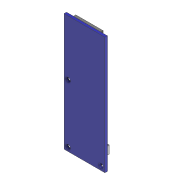
# Autodesk Inventor part: ESP32
Saved by Autodesk Inventor 2022.3 (Build 263350000, 350)
## iProperties
Created: 2023-07-18
Part Number: ESP32
Material: Genérico
Document SubType Name: Modeling
Designer: Usuario
Density: 1 g/cm^3
Appearance: Valor por defecto
Author: Usuario
Autodesk Inventor part; units mm, degrees
ref_plane "YZ Plane" through (0, 0, 0) normal (1, 0, 0) x (0, 1, 0)
ref_plane "XZ Plane" through (0, 0, 0) normal (0, 1, 0) x (-1, 0, 0)
ref_plane "XY Plane" through (0, 0, 0) normal (0, 0, 1) x (1, 0, 0)
sketch "Boceto1" plane through (0, 0, 0) normal (0, 0, 1) x (1, 0, 0)
  line L0 (-13.125, -37.65) -> (13.125, -37.65)
  line L1 (13.125, -37.65) -> (13.125, 37.65)
  line L2 (13.125, 37.65) -> (-13.125, 37.65)
  line L3 (-13.125, 37.65) -> (-13.125, -37.65)
  line L4 (-13.125, -37.65) -> (13.125, 37.65) construction
  line L5 (13.125, -37.65) -> (-13.125, 37.65) construction
  line L6 (0, -37.65) -> (0, -35.15)
  line L7 (0, -35.15) -> (10.5, -35.15)
  line L8 (10.5, -35.15) -> (-10.5, -35.15)
  circle A0 centre (10.5, -35.15) radius 1.5
  circle A1 centre (-10.5, -35.15) radius 1.5
  line L9 (-10.5, -35.15) -> (-10.5, 2.15)
  circle A2 centre (-10.5, 2.15) radius 1.5
  point P0 (0, 0)
  dimension "d0" = 26.25
  dimension "d1" = 75.3
  dimension "d2" = 2.5
  dimension "d3" = 10.5
  dimension "d4" = 21
  dimension "d5" = 3
  dimension "d6" = 3
  dimension "d7" = 37.3
  dimension "d8" = 3
  constraints: 20 end point, 3 centre point, 3 coincident, 3 midpoint, 3 perpendicular, 2 parallel, 1 horizontal, 1 point on line, 1 vertical
  measures "d0" distance of L2.end L1.end
  measures "d1" distance of L1.end L0.end
  measures "d2" distance of L6.start L6.end
  measures "d3" distance of L6.end L7.end
  measures "d4" distance of L7.end L8.end
  measures "d5" diameter of A0
  measures "d6" diameter of A1
  measures "d7" distance of L9.start L9.end
  measures "d8" diameter of A2
extrude "Extrusión1" add sketch "Boceto1" along normal blind 1.6
sketch "Boceto3" plane through (0, 0, 0) normal (0, 0, -1) x (-1, 0, 0)
  line L0 (-13.125, 37.65) -> (13.125, 37.65) projected
  line L1 (8.7698, 11.9975) -> (-8.7698, 11.9975)
  line L2 (-8.7698, 11.9975) -> (-8.7698, 37.65)
  line L3 (-8.7698, 37.65) -> (8.7698, 37.65)
  line L4 (8.7698, 37.65) -> (8.7698, 11.9975)
  line L5 (8.7698, 11.9975) -> (-8.7698, 37.65) construction
  line L6 (-8.7698, 11.9975) -> (8.7698, 37.65) construction
  line L7 (7.9072, -18.1146) -> (-7.9072, -18.1146)
  line L8 (-7.9072, -18.1146) -> (-7.9072, -2.2044)
  line L9 (-7.9072, -2.2044) -> (7.9072, -2.2044)
  line L10 (7.9072, -2.2044) -> (7.9072, -18.1146)
  line L11 (7.9072, -18.1146) -> (-7.9072, -2.2044) construction
  line L12 (-7.9072, -18.1146) -> (7.9072, -2.2044) construction
  point P0 (0, 0)
  point P1 (0, 24.8238)
  point P2 (0, -10.1595)
  constraints: 24 end point, 4 midpoint, 4 parallel, 2 horizontal, 2 perpendicular, 1 point on line
extrude "Extrusión2" add sketch "Boceto3" along normal blind 1.6
sketch "Boceto4" plane through (0, 0, -1.6) normal (0, 0, -1) x (-1, 0, 0)
  line L0 (8.003, 29.9035) -> (-8.003, 29.9035)
  line L1 (-8.003, 29.9035) -> (-8.003, 12.6515)
  line L2 (-8.003, 12.6515) -> (8.003, 12.6515)
  line L3 (8.003, 12.6515) -> (8.003, 29.9035)
  line L4 (8.003, 29.9035) -> (-8.003, 12.6515) construction
  line L5 (-8.003, 29.9035) -> (8.003, 12.6515) construction
  point P0 (0, 0)
  point P1 (0, 21.2775)
  constraints: 12 end point, 2 midpoint, 2 parallel, 1 horizontal, 1 perpendicular
extrude "Extrusión3" add sketch "Boceto4" along normal blind 2.5
sketch "Boceto5" plane through (-13.125, 37.65, 1.6) normal (0, 1, 0) x (1, 0, 0)
  line L0 (21.8948, 3.2) -> (4.3552, 3.2) projected
  line L1 (21.8948, 1.6) -> (21.8948, 3.2) projected
  line L2 (4.3552, 3.2) -> (21.8948, 3.2)
  line L3 (21.8948, 3.2) -> (21.8948, 1.6)
  line L4 (21.8948, 1.6) -> (4.3552, 1.6)
  line L5 (4.3552, 1.6) -> (4.3552, 3.2)
  point P0 (13.125, 1.6)
  constraints: 8 end point, 2 parallel, 1 horizontal, 1 perpendicular
extrude "Extrusión4" cut sketch "Boceto5" against normal blind 0.1
sketch "Boceto6" plane through (0, 0, -1.6) normal (0, 0, -1) x (-1, 0, 0)
  line L0 (5.9327, -11.7926) -> (-0.4732, -11.7926)
  line L1 (-0.4732, -11.7926) -> (-0.4732, -6.1147)
  line L2 (-0.4732, -6.1147) -> (5.9327, -6.1147)
  line L3 (5.9327, -6.1147) -> (5.9327, -11.7926)
  line L4 (5.9327, -11.7926) -> (-0.4732, -6.1147) construction
  line L5 (-0.4732, -11.7926) -> (5.9327, -6.1147) construction
  point P0 (0, 0)
  point P1 (2.7298, -8.9537)
  constraints: 12 end point, 2 midpoint, 2 parallel, 1 horizontal, 1 perpendicular
extrude "Extrusión5" add sketch "Boceto6" along normal blind 1
sketch "Boceto7" plane through (0, 0, 0) normal (0, 0, -1) x (-1, 0, 0)
  line L0 (13.125, 37.65) -> (13.125, -37.65) projected
  line L1 (13.125, -32.0293) -> (6.4423, -32.0293)
  line L2 (6.4423, -32.0293) -> (6.4423, -25.9874)
  line L3 (6.4423, -25.9874) -> (13.125, -25.9874)
  line L4 (13.125, -25.9874) -> (13.125, -32.0293)
  point P0 (0, 0)
  constraints: 8 end point, 2 parallel, 1 horizontal, 1 perpendicular, 1 point on line
extrude "Extrusión6" add sketch "Boceto7" along normal blind 5.5
sketch "Boceto8" plane through (0, 0, 0) normal (0, 0, -1) x (-1, 0, 0)
  line L0 (13.125, 37.65) -> (13.125, -37.65) projected
  line L1 (13.125, -25.3323) -> (9.5724, -25.3323)
  line L2 (9.5724, -25.3323) -> (9.5724, -19.5088)
  line L3 (9.5724, -19.5088) -> (13.125, -19.5088)
  line L4 (13.125, -19.5088) -> (13.125, -25.3323)
  line L5 (13.125, -37.65) -> (-13.125, -37.65) projected
  line L6 (-1.4923, -37.65) -> (-7.8981, -37.65)
  line L7 (-7.8981, -37.65) -> (-7.8981, -33.558)
  line L8 (-7.8981, -33.558) -> (-1.4923, -33.558)
  line L9 (-1.4923, -33.558) -> (-1.4923, -37.65)
  line L10 (-6.5151, -30.4279) -> (-11.3195, -30.4279)
  line L11 (-11.3195, -30.4279) -> (-11.3195, -25.3323)
  line L12 (-11.3195, -25.3323) -> (-6.5151, -25.3323)
  line L13 (-6.5151, -25.3323) -> (-6.5151, -30.4279)
  point P0 (0, 0)
  constraints: 24 end point, 6 parallel, 3 horizontal, 3 perpendicular, 2 point on line
extrude "Extrusión7" add sketch "Boceto8" along normal blind 3
sketch "Boceto9" plane through (-13.125, -37.65, 1.6) normal (0, -1, 0) x (1, 0, 0)
  line L0 (14.6173, -4.6) -> (21.0231, -4.6) projected
  line L1 (21.0231, -1.6) -> (21.0231, -4.6) projected
  line L2 (14.6173, -4.6) -> (21.0231, -4.6)
  line L3 (21.0231, -4.6) -> (21.0231, -1.6)
  line L4 (21.0231, -1.6) -> (14.6173, -1.6)
  line L5 (14.6173, -1.6) -> (14.6173, -4.6)
  point P0 (13.125, -1.6)
  constraints: 8 end point, 2 parallel, 1 horizontal, 1 perpendicular
extrude "Extrusión8" cut sketch "Boceto9" against normal blind 0.1
sketch "Boceto10" plane through (-13.125, -37.65, 1.6) normal (-1, 0, 0) x (0, 0, 1)
  line L0 (-4.6, 12.3177) -> (-4.6, 18.1412) projected
  line L1 (-1.6, 12.3177) -> (-1.6, 11.6626) projected
  line L2 (-4.6, 18.1412) -> (-1.6, 18.1412)
  line L3 (-1.6, 18.1412) -> (-1.6, 12.3177)
  line L4 (-1.6, 12.3177) -> (-4.6, 12.3177)
  line L5 (-4.6, 12.3177) -> (-4.6, 18.1412)
  line L6 (-7.1, 5.6207) -> (-7.1, 11.6626) projected
  line L7 (-1.6, 5.6207) -> (-7.1, 5.6207) projected
  line L8 (-7.1, 11.6626) -> (-1.6, 11.6626)
  line L9 (-1.6, 11.6626) -> (-1.6, 5.6207)
  line L10 (-1.6, 5.6207) -> (-7.1, 5.6207)
  line L11 (-7.1, 5.6207) -> (-7.1, 11.6626)
  point P0 (-1.6, 37.65)
  constraints: 16 end point, 4 parallel, 2 horizontal, 2 perpendicular
extrude "Extrusión9" cut sketch "Boceto10" against normal blind 0.1
